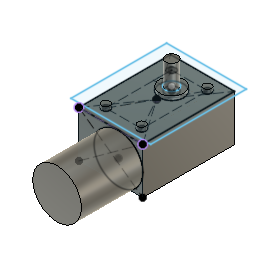
ButtonAxleLinearActuator v2 (Autodesk Fusion 360 archive; units mm, degrees)
design "Motor-JGY"
Autodesk Fusion 360 part; units mm, degrees
sketch "Mounting" plane through (0, 0, 0) normal (0, 0, 1) x (1, 0, 0)
  line L0 (9, -16.5) -> (-9, -16.5) construction
  line L1 (-9, -16.5) -> (-9, 16.5) construction
  line L2 (-9, 16.5) -> (9, 16.5) construction
  line L3 (9, 16.5) -> (9, -16.5) construction
  line L4 (9, -16.5) -> (-9, 16.5) construction
  line L5 (-9, -16.5) -> (9, 16.5) construction
  circle A0 centre (-9, 16.5) radius 2
  circle A1 centre (9, 16.5) radius 2
  circle A2 centre (9, -16.5) radius 2
  circle A3 centre (-9, -16.5) radius 2
  line L6 (16, -23) -> (-16, -23)
  line L7 (-16, -23) -> (-16, 23)
  line L8 (-16, 23) -> (16, 23)
  line L9 (16, 23) -> (16, -23)
  line L10 (16, -23) -> (-16, 23) construction
  line L11 (-16, -23) -> (16, 23) construction
  line L12 (-9, 16.5) -> (-9, 7.5) construction
  line L13 (-9, 7.5) -> (0, 7.5) construction
  circle A4 centre (0, 7.5) radius 6
  circle A5 centre (0, 7.5) radius 3
  dimension "d1" = 18
  dimension "d2" = 33
  dimension "d3" = 4
  dimension "d4" = 4
  dimension "d5" = 4
  dimension "d6" = 4
  dimension "d7" = 32
  dimension "d8" = 46
  dimension "d9" = 9
  dimension "d10" = 9
  dimension "d11" = 12
  dimension "d12" = 6
  constraint horizontal L0
  constraint perpendicular L0 L1
  constraint parallel L0 L2
  constraint parallel L1 L3
  constraint coincident L4 origin
  constraint coincident L5 origin
  constraint coincident L1.end L2.start
  constraint coincident L2.end L3.start
  constraint coincident L0.start L3.end
  constraint coincident L0.end L1.start
  constraint horizontal L6
  constraint perpendicular L6 L7
  constraint parallel L6 L8
  constraint parallel L7 L9
  constraint coincident L10 origin
  constraint coincident L11 origin
  constraint parallel L1 L12
  constraint perpendicular L12 L13
  constraint coincident L13.end A4.centre
  constraint concentric A4 A5
  measures "d1" distance of L1.end L2.end
  measures "d2" distance of L0.end L1.end
  measures "d3" diameter of A0
  measures "d4" diameter of A1
  measures "d5" diameter of A2
  measures "d6" diameter of A3
  measures "d7" distance of L7.end L8.end
  measures "d8" distance of L6.end L7.end
  measures "d9" distance of L1.end L12.end
  measures "d10" distance of L12.end L13.end
  measures "d11" diameter of A4
  measures "d12" diameter of A5
extrude "Extrude1" add sketch "Mounting" along normal blind 14 contours A5 makes body 1
extrude "Extrude2" add sketch "Mounting" along normal blind 2 contours A0 | A1 | A2 | A3 | A4 bodies 1 makes body 2 at (10.9975, -16.5997, 1.3333) makes body 3 at (10.9975, 16.4003, 1.3333) makes body 4 at (-7.0025, -16.5997, 1.3333) makes body 5 at (-7.0025, 16.4003, 1.3333)
extrude "Extrude3" add sketch "Mounting" against normal blind 25.2 separate body contours L6 L7 L8 L9 makes body 6
extrude "Extrude6" cut sketch "Mounting" against normal blind 29 contours L6 L7 L8 L9 bodies 6
extrude "Extrude7" add sketch "Mounting" against normal blind 23.2 contours L6 L7 L8 L9 bodies 6 1 2 3 4 5
sketch "Motor" plane through (0, -23, 0) normal (0, -1, 0) x (1, 0, 0)
  line L0 (16, 0) -> (-16, 0)
  line L1 (-16, 0) -> (-16, -23.2)
  line L2 (-16, -23.2) -> (16, -23.2)
  line L3 (16, -23.2) -> (16, 0)
  line L4 (-16, 0) -> (16, -23.2) construction
  line L5 (-16, -23.2) -> (16, 0) construction
  line L6 (16, 0) -> (-16, 0) construction
  circle A0 centre (3.8, -12.2) radius 12.2
  dimension "d29" = 12.2
  constraint coincident L0.end L1.start
  constraint coincident L2.end L3.start
  constraint coincident L1.end L2.start
  constraint coincident L0.start L3.end
  constraint tangent L3 A0
  constraint tangent L6 A0
  measures "d29" radius of A0
extrude "Extrude8" add sketch "Motor" along normal blind 30.8 separate body contours L2 A0 picked at (8.1727, -6.557) makes body 7
extrude "Extrude9" add sketch "Mounting" against normal blind 23.2 contours A0 | A1 | A2 | A3 | L6 L7 L8 L9 | A4 | A5 bodies 6 7
extrude "Extrude11" add sketch "Motor" along normal blind 30.8 contours L2 A0 picked at (4.9947, -23.4206) bodies 6
ref_plane "WorkPlane1" through (0, 0, 2) normal (0, 0, 1) x (1, 0, 0)
sketch "Sketch4" plane through (0, 0, 2) normal (0, 0, 1) x (1, 0, 0)
  line L0 (-20, 25) -> (20, 25)
  line L1 (20, 25) -> (20, -23)
  line L2 (20, -23) -> (-20, -23)
  line L3 (-20, -23) -> (-20, 25)
  circle A0 centre (0, 7.5) radius 3.25
  dimension "d39" = 6.5
  constraint horizontal L0
  constraint vertical L1
  constraint horizontal L2
  constraint vertical L3
  measures "d39" diameter of A0
extrude "Extrude10" [suppressed]
extrude "Extrude5" [suppressed]
extrude "Extrude4" [suppressed]
